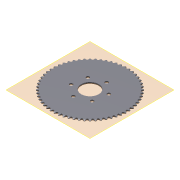
# Autodesk Inventor part: Roller Chain Sprocket1
Saved by Autodesk Inventor 2011 (Build 150239000, 239)
## iProperties
Created: 2012-05-18
Part Number: Roller Chain Sprocket1
Material: Steel
Document SubType Name: Modeling
Designer: niemitalo_dan
Density: 1 g/cm^3
CustomPartVersion: 1
Author: niemitalo_dan
Autodesk Inventor part; units mm, degrees
ref_plane "YZ Plane" through (0, 0, 0) normal (1, 0, 0) x (0, 1, 0)
ref_plane "XZ Plane" through (0, 0, 0) normal (0, 1, 0) x (-1, 0, 0)
sketch "Theoretical Tooth Profile" plane through (0, 0, 0) normal (0, 0, 1) x (1, 0, 0)
  circle A0 centre (0, 0) radius 60.6657 construction
  line L0 (0, 0) -> (0, 60.6657) construction
  line L1 (0, 0) -> (6.3413, 60.3334) construction
  circle A1 centre (0, 0) radius 62.4876
  arc A2 (-1.3482, 59.6862) -> (1.3482, 59.6862) centre (0, 60.6657) ccw
  line L2 (0, 60.6657) -> (6.3413, 60.3334) construction
  line L3 (0, 60.6657) -> (2.1358, 62.2175) construction
  line L4 (2.1358, 62.2175) -> (-1.9377, 60.8202) construction
  arc A3 (2.8583, 62.4222) -> (2.0978, 61.287) centre (4.6137, 60.424) ccw
  arc A4 (-2.0978, 61.287) -> (-2.8583, 62.4222) centre (-4.6137, 60.424) ccw
  line L5 (-4.6137, 60.424) -> (-2.0978, 61.287) construction
  arc A5 (-1.9377, 60.8202) -> (-1.3482, 59.6862) centre (2.1358, 62.2175) ccw
  line L6 (-1.9377, 60.8202) -> (-2.0978, 61.287)
  arc A6 (1.3482, 59.6862) -> (1.9377, 60.8202) centre (-2.1358, 62.2175) ccw
  line L7 (2.0978, 61.287) -> (1.9377, 60.8202)
  line L8 (0, 0) -> (3.2703, 62.402) construction
  point P0 (3.1706, 60.4996)
  dimension "d0" = 121.3315
  dimension "d2" = 6
  dimension "d3" = 1.6665
  dimension "d10" = 126
  dimension "d11" = 17.067
  dimension "d12" = 2.64
  dimension "d13" = 4.3065
  dimension "d14" = 4.62
  dimension "d23" = 1.905
  constraints: 18 end point, 15 point on circle, 7 centre point, 3 coincident, 3 point on line, 3 symmetric about line, 3 tangent, 1 equal radius, 1 midpoint, 1 parallel, 1 vertical, 1 other
  measures "d0" diameter of A0
  measures "d2" angle of L1 L0
  measures "d3" radius of A2
  measures "d10" angle of L3 L0
  measures "d11" angle of L4 L3
  measures "d12" distance of L2.start L3.end
  measures "d13" distance of L3.end L4.end
  measures "d14" distance of A3.centre L0.end
  measures "d23" distance from line of L8.end L2
sketch "Tooth Profile" plane through (0, 0, 0) normal (0, 0, 1) x (1, 0, 0)
  circle A0 centre (0, 0) radius 62.4876 projected
  line L0 (0, 0) -> (0, 60.6657) construction
  line L1 (0, 60.6657) -> (1.5584, 60.0753) construction
  arc A1 (-1.5584, 60.0753) -> (1.5584, 60.0753) centre (0, 60.6657) ccw
  line L2 (-1.5584, 60.0753) -> (0, 60.6657) construction
  arc A2 (-1.5584, 60.0753) -> (-2.5965, 62.4336) centre (-24.5178, 51.3768) ccw
  arc A3 (2.5965, 62.4336) -> (1.5584, 60.0753) centre (24.5178, 51.3768) ccw
  dimension "d44" = 138.5
  dimension "d45" = 1.6665
  dimension "d46" = 24.552
  constraints: 8 point on circle, 7 end point, 3 centre point, 2 tangent, 1 coincident, 1 equal radius, 1 symmetric about line, 1 vertical
  measures "d44" angle of L1 L2
  measures "d45" radius of A1
  measures "d46" radius of A3
sketch "Section Profile" plane through (0, 0, 0) normal (1, 0, 0) x (0, 1, 0)
  line L0 (62.4876, 0) -> (-62.4876, 0) projected
  line L1 (53.3982, 1.143) -> (-53.3982, 1.143)
  line L2 (-53.3982, 1.143) -> (-53.3982, -1.143)
  line L3 (-53.3982, -1.143) -> (53.3982, -1.143)
  line L4 (53.3982, -1.143) -> (53.3982, 1.143)
  line L5 (53.3982, 1.143) -> (62.4876, 1.143) construction
  line L6 (62.4876, 1.143) -> (62.4876, -1.143) construction
  line L7 (62.4876, -1.143) -> (53.3982, -1.143) construction
  line L8 (53.3982, -1.143) -> (53.3982, 1.143)
  arc A0 (62.4876, 0.3175) -> (59.3567, 1.143) centre (59.3567, -5.207) ccw
  arc A1 (59.3567, -1.143) -> (62.4876, -0.3175) centre (59.3567, 5.207) ccw
  line L9 (59.3567, 1.143) -> (0, 1.143)
  line L10 (0, 1.143) -> (0, -1.143)
  line L11 (0, -1.143) -> (59.3567, -1.143)
  line L12 (0, 1.143) -> (0, -1.143)
  line L13 (62.4876, 0.3175) -> (62.4876, -0.3175)
  point P0 (0, 0)
  point P1 (0, 0)
  dimension "d30" = 2.286
  dimension "d31" = 106.7964
  dimension "d32" = 2.286
  dimension "d33" = 0.8255
  dimension "d34" = 6.35
  dimension "d43" = 1.143
  constraints: 26 end point, 7 midpoint, 5 perpendicular, 4 parallel, 4 point on circle, 3 point on line, 3 symmetric about line, 2 centre point, 2 horizontal, 2 tangent, 1 collinear, 1 other
  measures "d30" distance between parallel lines of L7 L5
  measures "d31" distance between parallel lines of L2 L4
  measures "d32" distance between parallel lines of L3 L1
  measures "d33" distance from line of L13.start L5
  measures "d34" radius of A0
  measures "d43" distance between parallel lines of L3 L0
revolve "Shroud" add sketch "Section Profile" angle 360 about axis through (0, 0, 1.143) along (0, 0, -1) contours L10 L3 L2 L0 | L0 L2 L1 L10
revolve "Strand" add sketch "Section Profile" angle 360 about axis through (0, 0, 1.143) along (0, 0, -1) contours L13 A1 L11 L4 L0 | L0 L4 L9 A0 L13 | L4 L3 L10 L0 | L0 L10 L1 L4
pattern_of_one "Strand Pattern"
extrude "Theoretical Tooth" cut sketch "Theoretical Tooth Profile" along normal through all both and the other way through all contours A3 L7 A6 A2 A5 L6 A4 A1 picked at (-0.3177, 60.8561)
extrude "Tooth" [suppressed]
pattern_circular "Tooth Pattern" count 60 over 360 about axis through (0, 0, -10) along (0, 0, 1) of "Theoretical Tooth"
ref_plane "Timing Plane" through (0, 60.6657, 0) normal (1, 0, 0) x (0, 1, 0)
sketch "Sketch4" plane through (0, 0, 1.143) normal (0, 0, 1) x (0.9986295, -0.052336, 0)
  arc A0 (8.2765, 58.7769) -> (4.1248, 59.2132) centre (0, 0) ccw projected
  circle A1 centre (0, 0) radius 14.2875
  dimension "d51" = 28.575
  constraints: 1 centre point, 1 coincident
  measures "d51" diameter of A1
extrude "Extrusion4" cut sketch "Sketch4" against normal through all
sketch "Sketch5" plane through (0, 0, -1.143) normal (0, 0, -1) x (-0.9876883, 0.1564345, 0)
  circle A0 centre (0, 0) radius 14.2875 projected
  point P0 (0, 23.8125)
  point P1 (-20.6222, 11.9063)
  point P2 (-20.6222, -11.9062)
  point P3 (0, -23.8125)
  point P4 (20.6222, -11.9063)
  point P5 (20.6222, 11.9062)
  dimension "d54" = 23.8125
  dimension "d57" = 360
  constraints: 7 other
  measures "d54" distance of A0.centre point (0, 23.812)
hole "Hole1" at (3.7251, 23.5193, -1.143) at (22.2309, 8.5336, -1.143) at (18.5058, -14.9857, -1.143) at (-3.7251, -23.5193, -1.143) at (-22.2309, -8.5336, -1.143) at (-18.5058, 14.9857, -1.143) direction (0, 0, 1) diameter 5.2324 end through all
equation "\"d3\" = 0.5 * da_Dr + da_SC"
equation "\"d12\" = 0.8 * da_Dr"
equation "\"d13\" = 1.3 * da_Dr + da_SC"
equation "\"d14\" = 1.4 * da_Dr"
equation "\"d23\" = da_Ha"
equation "\"d44\" = da_Alfa"
equation "\"d45\" = da_Ri"
equation "\"d46\" = da_Re"
equation "\"d30\" = da_Bf"
equation "\"d31\" = da_Ds"
equation "\"d32\" = da_Bs"
equation "\"d33\" = da_Ba"
equation "\"d34\" = da_Rx"
equation "\"d40\" = da_pt"
equation "\"form_type\" = 0"
equation "\"da_p\" = 6.35"
equation "\"da_Dr\" = 3.3"
equation "\"da_SC\" = 0.0165"
equation "\"da_Ha\" = 1.905"
equation "\"da_pt\" = 6.4"
equation "\"da_Bf\" = 2.286"
equation "\"da_Ba\" = 0.8255"
equation "\"da_Rx\" = 6.35"
equation "\"da_Ra\" = 0.254"
equation "\"da_Bs\" = 2.286"
equation "\"da_Ds\" = 106.79642"
equation "\"da_Re\" = 24.552"
equation "\"da_Ri\" = 1.6665"
equation "\"da_Alfa\" = 138.5deg"
body "Solid1"
